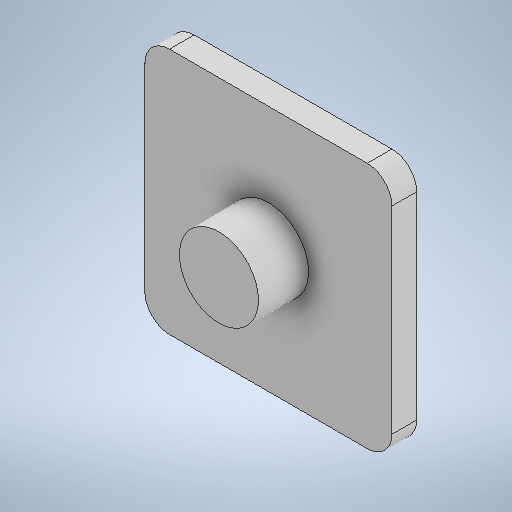
# Autodesk Inventor part: Base2
Saved by Autodesk Inventor 2025.2 (Build 292293000, 293)
## iProperties
Created: 2025-03-03
Part Number: Base2
Material: Generic
Document SubType Name: Modeling
Designer: Marcu
Density: 1 g/cm^3
Appearance: Default
Author: Marcu
Autodesk Inventor part; units mm, degrees
ref_plane "YZ Plane" through (0, 0, 0) normal (1, 0, 0) x (0, 1, 0)
ref_plane "XZ Plane" through (0, 0, 0) normal (0, 1, 0) x (-1, 0, 0)
ref_plane "XY Plane" through (0, 0, 0) normal (0, 0, 1) x (1, 0, 0)
sketch "Sketch1" plane through (0, 0, 0) normal (0, 1, 0) x (-1, 0, 0)
  line L0 (25, 25) -> (-25, 25)
  line L1 (-25, 25) -> (-25, -25)
  line L2 (-25, -25) -> (25, -25)
  line L3 (25, -25) -> (25, 25)
  point P0 (0, 0)
  dimension "d0" = 50
  dimension "d1" = 50
  dimension "d2" = 25
  dimension "d3" = 25
  constraints: 8 end point, 2 parallel, 1 horizontal, 1 perpendicular
  measures "d0" distance between parallel lines of L2 L0
  measures "d1" distance between parallel lines of L1 L3
  measures "d2" distance from line of point (0, 0) L2
  measures "d3" distance from line of point (0, 0) L1
extrude "Extrusion1" add sketch "Sketch1" along normal blind 5
sketch "Sketch2" plane through (0, 0, 0) normal (0, -1, 0) x (1, 0, 0)
  circle A0 centre (0, 0) radius 8
  dimension "d6" = 16
  constraints: 1 centre point, 1 coincident
  measures "d6" diameter of A0
extrude "Extrusion2" add sketch "Sketch2" along normal blind 10
sketch "Sketch3" plane through (0, 5, 0) normal (0, 1, 0) x (1, 0, 0)
  line L0 (0, -3) -> (0, -3)
  line L1 (3, 0) -> (3, 0)
  line L2 (0, 3) -> (0, 3)
  line L3 (-3, 0) -> (-3, 0)
  arc A0 (-3, 0) -> (0, -3) centre (0, 0) ccw
  arc A1 (0, 3) -> (-3, 0) centre (0, 0) ccw
  arc A2 (3, 0) -> (0, 3) centre (0, 0) ccw
  arc A3 (0, -3) -> (3, 0) centre (0, 0) ccw
  point P0 (0, 0)
  dimension "d9" = 6
  dimension "d10" = 6
  dimension "d11" = 3
  dimension "d12" = 3
  dimension "d19" = 3
  constraints: 8 end point, 8 point on circle, 8 tangent, 4 centre point, 3 concentric, 2 parallel, 1 horizontal, 1 perpendicular
  measures "d9" distance between parallel lines of L0 L2
  measures "d10" distance between parallel lines of L1 L3
  measures "d11" distance from line of point (0, 0) L0
  measures "d12" distance from line of point (0, 0) L1
  measures "d19" radius of A0
extrude "Extrusion3" cut sketch "Sketch3" against normal blind 6
sketch "Sketch4" plane through (0, 5, 0) normal (0, 1, 0) x (1, 0, 0)
  line L0 (-5, -5) -> (-5, 5) projected
  line L1 (-25, 25) -> (-25, -25) projected
  circle A0 centre (-15, 0) radius 2.5
  line L2 (5, -5) -> (-5, -5) projected
  line L3 (-5, 5) -> (5, 5) projected
  circle A1 centre (15, 0) radius 2.5
  line L4 (25, -25) -> (25, 25) projected
  point P0 (0, 0)
  dimension "d15" = 5
  dimension "d20" = 10
  dimension "d21" = 10
  constraints: 2 centre point
  measures "d15" diameter of A0
  measures "d20" distance from line of L1 A0.centre
  measures "d21" distance from line of A1.centre L4
extrude "Extrusion4" cut sketch "Sketch4" against normal blind 3
fillet "Fillet1" radius 5 4 edges at (25, 2.5, 25) (25, 2.5, -25) (-25, 2.5, -25) (-25, 2.5, 25)
sketch "Sketch5" plane through (0, 0, 0) normal (1, 0, 0) x (0, 1, 0)
  line L0 (0, 8) -> (-10, 8) projected
  line L1 (0, 8) -> (0, 8.125)
  line L2 (0, 20) -> (0, -20) projected
  line L3 (-10, 8) -> (-10, -8) projected
  line L4 (0, 8.125) -> (-10, 8)
  line L5 (-10, 8) -> (0, 8)
  line L6 (-10, 0) -> (0, 0)
  dimension "d23" = 0.125
  constraints: 8 end point, 2 point on line, 1 horizontal, 1 midpoint, 1 perpendicular
  measures "d23" distance of L1.start L1.end
revolve "Revolution1" add sketch "Sketch5" angle 360 about axis through (0, -10, 0) along (0, 1, 0) contours L0 L4 L1
body "Solid1"
